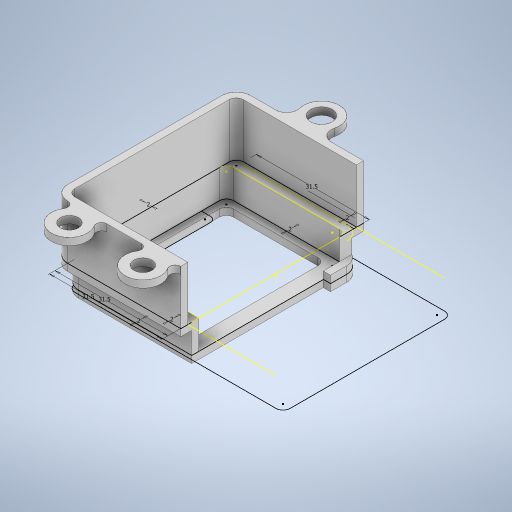
# Autodesk Inventor part: CO-1-01-motorControllersMount
Saved by Autodesk Inventor 2023 (Build 270158000, 158)
## iProperties
Created: 2023-01-24
Part Number: CO-1-01-motorControllersMount
Material: Generic
Document SubType Name: Modeling
Designer: t205b
Density: 1 g/cm^3
Appearance: Default
Author: t205b
Autodesk Inventor part; units mm, degrees
ref_plane "YZ Plane" through (0, 0, 0) normal (1, 0, 0) x (0, 1, 0)
ref_plane "XZ Plane" through (0, 0, 0) normal (0, 1, 0) x (-1, 0, 0)
sketch "Sketch1" plane through (0, 0, 0) normal (0, 1, 0) x (-1, 0, 0)
  arc A0 (31.569, 13.7227) -> (30.069, 12.2227) centre (31.569, 12.2227) ccw
  line L0 (31.569, 13.7227) -> (34.069, 13.7227)
  line L1 (34.069, 13.7227) -> (34.069, 18.9227)
  line L2 (32.069, 20.9227) -> (0.569, 20.9227)
  line L3 (-1.431, -13.7773) -> (0.569, -13.7773)
  line L4 (0.569, -13.7773) -> (0.569, -18.2773)
  line L5 (34.069, -13.2773) -> (31.569, -13.2773)
  arc A1 (30.069, -11.7773) -> (31.569, -13.2773) centre (31.569, -11.7773) ccw
  arc A2 (34.069, 18.9227) -> (32.069, 20.9227) centre (32.069, 18.9227) ccw
  arc A3 (34.0195, 22.4149) -> (32.069, 23.9727) centre (32.069, 21.9727) ccw
  line L6 (32.069, 23.9727) -> (-23.931, 23.9727)
  arc A4 (-23.931, 23.9727) -> (-25.931, 21.9727) centre (-23.931, 21.9727) ccw
  line L7 (-25.931, 21.9727) -> (-25.931, -21.0273)
  arc A5 (-25.931, -21.0273) -> (-23.931, -23.0273) centre (-23.931, -21.0273) ccw
  line L8 (-23.931, -23.0273) -> (32.069, -23.0273)
  arc A6 (32.069, -23.0273) -> (33.899, -21.8341) centre (32.069, -21.0273) ccw
  arc A7 (32.069, -20.2773) -> (34.069, -18.2773) centre (32.069, -18.2773) ccw
  line L9 (32.069, -20.2773) -> (2.569, -20.2773)
  arc A8 (0.569, -18.2773) -> (2.569, -20.2773) centre (2.569, -18.2773) ccw
  line L10 (34.069, -13.2773) -> (34.069, 13.7227)
  line L11 (0.569, -13.7773) -> (0.569, 20.9227)
  line L12 (30.069, -11.7773) -> (30.069, 12.2227)
  line L13 (0.569, 22.9227) -> (0.569, 20.9227)
  line L14 (34.069, -18.2773) -> (34.069, -13.2773)
  line L15 (0.569, 22.9227) -> (32.069, 22.9227)
  arc A9 (36.069, 18.9227) -> (32.069, 22.9227) centre (32.069, 18.9227) ccw
  line L16 (-1.431, -13.7773) -> (-1.431, -18.2773)
  arc A10 (-1.431, -18.2773) -> (2.569, -22.2773) centre (2.569, -18.2773) ccw
  line L17 (2.569, -22.2773) -> (32.069, -22.2773)
  arc A11 (32.069, -22.2773) -> (36.069, -18.2773) centre (32.069, -18.2773) ccw
  line L18 (36.069, -18.2773) -> (36.069, 18.9227)
  dimension "d8" = 2
  dimension "d9" = 2
  constraints: 40 end point, 27 point on circle, 12 centre point, 10 vertical, 8 horizontal, 1 collinear, 1 perpendicular, 13 other
  measures "d8" distance between parallel lines of L2 L15
  measures "d9" distance between parallel lines of L9 L17
extrude "Extrusion3" add sketch "Sketch1" against normal blind 2 contours L0 L10 L5 A1 L12 A0 | A0 L12 A1 L5 L14 A7 L9 A8 L4 L11 L2 A2 L1 L0 | L1 A2 L2 L13 L15 A9 L18 A11 L17 A10 L16 L3 L4 A8 L9 A7 L14 L10
ref_plane "Work Plane1" through (0, 8, 0) normal (0, 1, 0) x (1, 0, 0)
extrude "Extrusion4" add sketch "Sketch1" along normal blind 8 contours L1 A2 L2 L13 L15 A9 L18 A11 L17 A10 L16 L3 L4 A8 L9 A7 L14 L10
sketch "Sketch2" plane through (0, 8, 0) normal (0, 1, 0) x (1, 0, 0)
  line L0 (23.931, 23.0273) -> (-32.069, 23.0273) projected
  arc A0 (-32.069, 23.0273) -> (-33.899, 21.8341) centre (-32.069, 21.0273) ccw projected
  line L1 (-32.069, -23.9727) -> (23.931, -23.9727) projected
  arc A1 (-34.0195, -22.4149) -> (-32.069, -23.9727) centre (-32.069, -21.9727) ccw projected
  line L2 (-36.069, 18.2773) -> (-36.069, -18.9227) projected
  arc A2 (-32.069, 23.0273) -> (-34.069, 21.0273) centre (-32.069, 21.0273) ccw
  arc A3 (-34.069, -21.9727) -> (-32.069, -23.9727) centre (-32.069, -21.9727) ccw
  line L3 (-34.069, 18.2773) -> (-34.069, 13.2773) projected
  line L4 (-34.069, 13.2773) -> (-34.069, -13.7227) projected
  line L5 (-34.069, -13.7227) -> (-34.069, -18.9227) projected
  line L6 (-34.069, -21.9727) -> (-34.069, 21.0273)
  arc A4 (-32.069, 25.0273) -> (-36.069, 21.0273) centre (-32.069, 21.0273) ccw
  line L7 (-36.069, 21.0273) -> (-36.069, -21.9727)
  arc A5 (-36.069, -21.9727) -> (-32.069, -25.9727) centre (-32.069, -21.9727) ccw
  line L8 (-0.569, 25.0273) -> (-32.069, 25.0273)
  arc A6 (-32.069, 25.0273) -> (-35.729, 22.6409) centre (-32.069, 21.0273) ccw
  line L9 (-0.569, -25.9727) -> (-32.069, -25.9727)
  arc A7 (-35.97, -22.8571) -> (-32.069, -25.9727) centre (-32.069, -21.9727) ccw
  line L10 (-0.569, 13.7773) -> (-0.569, -22.9227) projected
  line L11 (-0.569, -23.9727) -> (-0.569, -25.9727)
  line L12 (-0.569, 18.2773) -> (-0.569, 25.0273)
  line L13 (-0.569, 13.7773) -> (-0.569, 18.2773) projected
  line L14 (-32.069, 23.0273) -> (-0.569, 23.0273)
  line L15 (-32.069, -23.9727) -> (-0.569, -23.9727)
  arc A8 (-0.569, 18.2773) -> (-2.569, 20.2773) centre (-2.569, 18.2773) ccw projected
  line L16 (-32.069, -20.9227) -> (-0.569, -20.9227) projected
  line L17 (-0.569, -20.9227) -> (-0.569, 13.7773) projected
  line L18 (-0.569, 13.7773) -> (-0.569, 18.2773) projected
  arc A9 (-0.569, 18.2773) -> (-2.569, 20.2773) centre (-2.569, 18.2773) ccw projected
  line L19 (-2.569, 20.2773) -> (-32.069, 20.2773) projected
  arc A10 (-32.069, 20.2773) -> (-34.069, 18.2773) centre (-32.069, 18.2773) ccw projected
  line L20 (-34.069, 18.2773) -> (-34.069, -18.9227) projected
  arc A11 (-34.069, -18.9227) -> (-32.069, -20.9227) centre (-32.069, -18.9227) ccw projected
  line L21 (-0.569, -23.9727) -> (-0.569, -22.9227)
  line L22 (-32.069, 22.2773) -> (-2.569, 22.2773) projected
  line L23 (-2.569, 22.2773) -> (-0.569, 22.2773)
  arc A12 (1.431, 18.2773) -> (-2.569, 22.2773) centre (-2.569, 18.2773) ccw projected
  point P0 (0, 0)
  point P1 (-0.569, 21.7414)
  dimension "d18" = 2
  dimension "d19" = 2
  dimension "d20" = 2
  dimension "d21" = 31.5
  dimension "d22" = 31.5
  dimension "d23" = 31.5
  constraints: 22 end point, 13 point on circle, 6 centre point, 6 point on line, 4 perpendicular, 2 coincident, 2 tangent, 2 vertical, 1 concentric, 1 horizontal, 2 other
  measures "d18" distance between parallel lines of L6 L7
  measures "d19" distance between parallel lines of L0 L8
  measures "d20" distance between parallel lines of L1 L9
  measures "d21" distance of L9.start L9.end
  measures "d22" distance of L1.start L11.start
  measures "d23" distance of L8.start L8.end
sketch "Sketch3" plane through (0, 8, 0) normal (0, 1, 0) x (1, 0, 0)
  line L0 (-0.569, 18.2773) -> (-0.569, 13.7773) projected
  line L1 (-0.569, 13.7773) -> (1.431, 13.7773) projected
  line L2 (1.431, 13.7773) -> (1.431, 18.2773) projected
  arc A0 (1.431, 18.2773) -> (-2.569, 22.2773) centre (-2.569, 18.2773) ccw projected
  line L3 (-0.569, -20.9227) -> (-32.069, -20.9227) projected
  arc A1 (-34.069, -18.9227) -> (-32.069, -20.9227) centre (-32.069, -18.9227) ccw projected
  line L4 (-34.069, -18.9227) -> (-34.069, 18.2773) projected
  arc A2 (-32.069, 20.2773) -> (-34.069, 18.2773) centre (-32.069, 18.2773) ccw projected
  line L5 (-32.069, 20.2773) -> (-2.569, 20.2773) projected
  arc A3 (-0.569, 18.2773) -> (-2.569, 20.2773) centre (-2.569, 18.2773) ccw projected
  arc A4 (-32.069, 22.2773) -> (-36.069, 18.2773) centre (-32.069, 18.2773) ccw projected
  line L6 (-36.069, 18.2773) -> (-36.069, -18.9227) projected
  arc A5 (-36.069, -18.9227) -> (-32.069, -22.9227) centre (-32.069, -18.9227) ccw projected
  line L7 (-32.069, -22.9227) -> (-0.569, -22.9227) projected
  line L8 (-0.569, -22.9227) -> (-0.569, -20.9227) projected
  line L9 (-2.569, 22.2773) -> (-32.069, 22.2773) projected
  point P0 (0, 0)
extrude "Extrusion7" add sketch "Sketch2" against normal blind 2 contours L12 L23 A12 A8 L19 A10 L6 A2 A0 L0 | L0 A0 A2 L6 L3 L4 L5 A3 A1 L1 L11 L9 A5 L7 L2 A4 L8 L12 | L12 A12 L23 | L10 L21 L1 A1 A3 L6 A11 L16
extrude "Extrusion8" add sketch "Sketch2" along normal blind 15 contours L0 A0 A2 L6 L3 L4 L5 A3 A1 L1 L11 L9 A5 L7 L2 A4 L8 L12
sketch "Sketch4" plane through (0, 8, 0) normal (0, 1, 0) x (1, 0, 0)
  line L0 (1.431, 13.7773) -> (1.431, 18.2773) projected
  line L1 (-0.569, 13.7773) -> (1.431, 13.7773) projected
  line L2 (-0.569, 18.2773) -> (-0.569, 25.0273) projected
  line L3 (-0.569, 18.2773) -> (-0.569, 13.7773) projected
  arc A0 (1.431, 18.2773) -> (-0.569, 21.7414) centre (-2.569, 18.2773) ccw projected
  point P0 (0, 0)
extrude "Extrusion9" cut sketch "Sketch4" against normal blind 6
sketch "Sketch5" plane through (0, 23, 0) normal (0, 1, 0) x (1, 0, 0)
  circle A0 centre (-17.319, 30.0273) radius 5
  circle A1 centre (-17.319, 30.0273) radius 3
  line L0 (-0.569, 25.0273) -> (-32.069, 25.0273) projected
  arc A2 (-12.4777, 28.7773) -> (-9.573, 25.0273) centre (-9.573, 28.0273) ccw
  arc A3 (-25.0649, 25.0273) -> (-22.1602, 28.7773) centre (-25.0649, 28.0273) ccw
  line L1 (-0.569, 23.0273) -> (-0.569, 25.0273) projected
  line L2 (-34.069, -21.9727) -> (-34.069, 21.0273) projected
  circle A4 centre (-6.0917, -30.9727) radius 5
  circle A5 centre (-6.0917, -30.9727) radius 2.5
  arc A6 (-10.305, -28.2804) -> (-11.569, -25.9727) centre (-11.569, -27.4727) ccw
  arc A7 (-0.6145, -25.9727) -> (-1.8785, -28.2804) centre (-0.6145, -27.4727) ccw
  line L3 (-32.069, -25.9727) -> (-0.569, -25.9727) projected
  circle A8 centre (-26.5917, -30.9727) radius 5
  circle A9 centre (-26.5917, -30.9727) radius 2.5
  arc A10 (-30.805, -28.2804) -> (-32.069, -25.9727) centre (-32.069, -27.4727) ccw
  arc A11 (-21.1145, -25.9727) -> (-22.3785, -28.2804) centre (-21.1145, -27.4727) ccw
  line L4 (-0.569, -25.9727) -> (-0.569, -23.9727) projected
  arc A12 (-36.069, -21.9727) -> (-32.069, -25.9727) centre (-32.069, -21.9727) ccw projected
  point P0 (0, 0)
  point P1 (1.0185, -24.3852)
  dimension "d34" = 10
  dimension "d35" = 6
  dimension "d36" = 33.5
  dimension "d37" = 16.75
  dimension "d38" = 3
  dimension "d39" = 3
  dimension "d40" = 10
  dimension "d41" = 5
  dimension "d42" = 3
  dimension "d43" = 3
  dimension "d44" = 10
  dimension "d45" = 5
  dimension "d46" = 3
  dimension "d47" = 3
  dimension "d49" = 20.5
  constraints: 18 point on circle, 16 tangent, 12 centre point, 6 point on line, 3 coincident
  measures "d34" diameter of A0
  measures "d35" diameter of A1
  measures "d36" distance between parallel lines of L1 L2
  measures "d37" distance from line of A0.centre L2
  measures "d38" radius of A3
  measures "d39" radius of A2
  measures "d40" diameter of A4
  measures "d41" diameter of A5
  measures "d42" diameter of A6
  measures "d43" diameter of A7
  measures "d44" diameter of A8
  measures "d45" diameter of A9
  measures "d46" diameter of A10
  measures "d47" diameter of A11
  measures "d49" distance of A4.centre A8.centre
extrude "Extrusion10" add sketch "Sketch5" against normal blind 2
sketch "Sketch6" plane through (0, -2, 0) normal (0, -1, 0) x (1, 0, 0)
  line L0 (1.431, -18.2773) -> (1.431, -13.7773) projected
  line L1 (1.431, -13.7773) -> (-0.569, -13.7773) projected
  line L2 (-0.569, -13.7773) -> (-0.569, 22.9227) projected
  line L3 (-0.569, 22.9227) -> (-32.069, 22.9227) projected
  arc A0 (-32.069, 22.9227) -> (-36.069, 18.9227) centre (-32.069, 18.9227) ccw projected
  line L4 (-36.069, 18.9227) -> (-36.069, -18.2773) projected
  arc A1 (-36.069, -18.2773) -> (-32.069, -22.2773) centre (-32.069, -18.2773) ccw projected
  line L5 (-32.069, -22.2773) -> (-2.569, -22.2773) projected
  arc A2 (-2.569, -22.2773) -> (1.431, -18.2773) centre (-2.569, -18.2773) ccw projected
  line L6 (-30.069, 18.9227) -> (-6.569, 18.9227)
  line L7 (-4.569, 16.9227) -> (-4.569, -16.2773)
  line L8 (-6.569, -18.2773) -> (-30.069, -18.2773)
  line L9 (-32.069, -16.2773) -> (-32.069, 16.9227)
  arc A3 (-6.569, -18.2773) -> (-4.569, -16.2773) centre (-6.569, -16.2773) ccw
  arc A4 (-32.069, -16.2773) -> (-30.069, -18.2773) centre (-30.069, -16.2773) ccw
  arc A5 (-30.069, 18.9227) -> (-32.069, 16.9227) centre (-30.069, 16.9227) ccw
  arc A6 (-4.569, 16.9227) -> (-6.569, 18.9227) centre (-6.569, 16.9227) ccw
  point P0 (0, 0)
  point P1 (-4.569, 18.9227)
  point P2 (-4.569, -18.2773)
  dimension "d52" = 4
  dimension "d53" = 37.2
  dimension "d54" = 27.5
  dimension "d55" = 4
  dimension "d56" = 2
  constraints: 8 end point, 8 point on circle, 8 tangent, 4 centre point, 4 point on line, 3 equal radius, 3 perpendicular
  measures "d52" distance between parallel lines of L3 L6
  measures "d53" distance of point (-4.569, 18.923) point (-4.569, -18.277)
  measures "d54" distance between parallel lines of L7 L9
  measures "d55" distance between parallel lines of L2 L7
  measures "d56" radius of A3
extrude "Extrusion11" cut sketch "Sketch6" against normal blind 2 contours L6 A6 L7 A3 L8 A4 L9 A5
equation "\"d37\" = 0.5 * d36"
body "Solid2"
